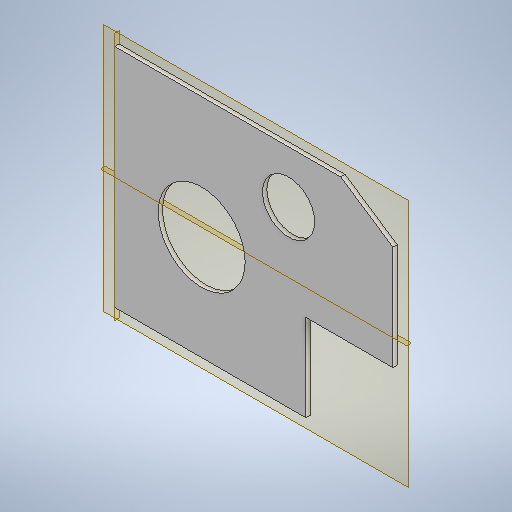
# Autodesk Inventor part: chap2ex2
Saved by Autodesk Inventor 2025.2 (Build 292293000, 293)
## iProperties
Created: 2025-01-31
Part Number: chap2ex2
Material: Generic
Document SubType Name: Modeling
Designer: Moofin
Density: 1 g/cm^3
Appearance: Default
Author: Moofin
Autodesk Inventor part; units mm, degrees
sketch "Sketch1" plane through (0, 0, 0) normal (0, 0, 1) x (1, 0, 0)
  line L0 (0, 82.55) -> (203.2, 82.55)
  line L1 (203.2, 82.55) -> (203.2, -82.55)
  line L2 (203.2, -82.55) -> (0, -82.55)
  line L3 (0, -82.55) -> (0, 82.55)
  line L4 (0, 115.57) -> (0, -115.57) projected
  line L5 (-40.64, 0) -> (243.84, 0) projected
  point P0 (0, 0)
  dimension "d0" = 0
  dimension "d1" = 165.1
  dimension "d2" = 203.2
  dimension "d3" = 82.55
  constraints: 8 end point, 2 parallel, 1 horizontal, 1 perpendicular
  measures "d0" distance between parallel lines of L4 L3
  measures "d1" distance between parallel lines of L2 L0
  measures "d2" distance between parallel lines of L1 L3
  measures "d3" distance between parallel lines of L5 L0
extrude "Extrusion1" add sketch "Sketch1" along normal mid plane 3.175
sketch "Sketch2" plane through (0, 0, 1.5875) normal (0, 0, 1) x (1, 0, 0)
  circle A0 centre (127, 44.45) radius 19.05
  line L0 (0, 82.55) -> (0, -82.55) projected
  line L1 (203.2, 82.55) -> (0, 82.55) projected
  circle A1 centre (63.5, -6.35) radius 31.75
  line L2 (0, -82.55) -> (203.2, -82.55) projected
  line L3 (203.2, -82.55) -> (203.2, 82.55) projected
  line L4 (203.2, -19.05) -> (139.7, -19.05)
  line L5 (139.7, -19.05) -> (139.7, -82.55)
  point P0 (0, 0)
  dimension "d6" = 38.1
  dimension "d7" = 127
  dimension "d8" = 38.1
  dimension "d9" = 63.5
  dimension "d10" = 63.5
  dimension "d11" = 76.2
  dimension "d14" = 63.5
  dimension "d15" = 63.5
  constraints: 4 end point, 2 centre point, 2 point on line, 1 horizontal, 1 perpendicular
  measures "d6" diameter of A0
  measures "d7" distance from line of L0 A0.centre
  measures "d8" distance from line of L1 A0.centre
  measures "d9" diameter of A1
  measures "d10" distance from line of L0 A1.centre
  measures "d11" distance from line of L2 A1.centre
  measures "d14" distance of L4.start L4.end
  measures "d15" distance between parallel lines of L2 L4
extrude "Extrusion2" cut sketch "Sketch2" against normal up to surface (3.175 mm away) contours A0 | L5 L4 L3 L2 | A1
chamfer "Chamfer1" distance 25.4 distance2 38.1 1 edges at (203.2, 82.55, 0) measured on face at (203.2, 14.8167, -0.5292)
equation "\"d3\" = 0.5 * d1"
body "Solid1"
